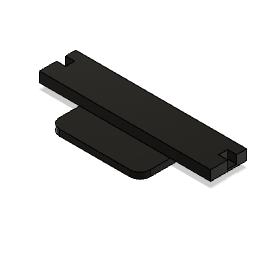
closing_electronic_box (Autodesk Fusion 360 design; units mm, degrees)
Autodesk Fusion 360 part; units mm, degrees
note: some values were not read from the file. Set by a fixed rule: which sketch regions a step uses.
sketch "Esquisse1" plane through (0, 0, 0) normal (0, 1, 0) x (1, 0, 0)
  line L0 (-42.5, 9) -> (42.5, 9)
  line L1 (42.5, 9) -> (42.5, -9)
  line L2 (42.5, -9) -> (-42.5, -9)
  line L3 (-42.5, -9) -> (-42.5, 9)
  line L4 (-42.5, 9) -> (42.5, -9) construction
  line L5 (42.5, 9) -> (-42.5, -9) construction
  dimension "d1" = 18
  dimension "d2" = 85
  constraint horizontal L0
  constraint perpendicular L0 L1
  constraint parallel L0 L2
  constraint parallel L1 L3
  constraint coincident L4 origin
  constraint coincident L5 origin
  measures "d1" distance of L0.start L2.end
  measures "d2" distance of L1.end L2.end
extrude "Extrusion1" add sketch "Esquisse1" along normal blind 5
sketch "Esquisse2" plane through (0, 5, 0) normal (0, 1, 0) x (-1, 0, 0)
  line L0 (42.5, 9) -> (-42.5, 9)
  line L1 (-42.5, 9) -> (-42.5, -9)
  line L2 (-42.5, -9) -> (42.5, -9)
  line L3 (42.5, -9) -> (42.5, 9)
  line L4 (42.5, -4) -> (38, -4)
  line L5 (38, -4) -> (38, 0.5)
  line L6 (38, 0.5) -> (42.5, 0.5)
  line L7 (42.5, 0.5) -> (42.5, -4)
  line L8 (-42.5, -4) -> (-38, -4)
  line L9 (-38, -4) -> (-38, 0.5)
  line L10 (-38, 0.5) -> (-42.5, 0.5)
  line L11 (-42.5, 0.5) -> (-42.5, -4)
  dimension "d5" = 5
  dimension "d6" = 4.5
  dimension "d7" = 4.5
  dimension "d8" = 5
  dimension "d9" = 4.5
  dimension "d10" = 4.5
  constraint horizontal L4
  constraint vertical L5
  constraint horizontal L6
  constraint vertical L7
  constraint coincident L3 L4.start
  constraint horizontal L8
  constraint vertical L9
  constraint horizontal L10
  constraint vertical L11
  constraint coincident L1 L8.start
  measures "d5" distance of L2 L4
  measures "d6" distance of L4.end L5.end
  measures "d7" distance of L5.end L6.end
  measures "d8" distance of L2 L8
  measures "d9" distance of L8.start L8.end
  measures "d10" distance of L8.end L9.end
extrude "Extrusion2" cut sketch "Esquisse2" against normal blind 4 contours L3 L4 L5 L6 L7 | L1 L8 L9 L10 L11
sketch "Esquisse3" plane through (0, 0, 0) normal (0, -1, 0) x (1, 0, 0)
  line L0 (42.5, 9) -> (-42.5, 9)
  line L1 (-42.5, 9) -> (-42.5, -9)
  line L2 (-42.5, -9) -> (42.5, -9)
  line L3 (42.5, -9) -> (42.5, 9)
  line L4 (-15, 5) -> (15, 5)
  line L5 (15, 5) -> (15, -5)
  line L6 (15, -5) -> (-15, -5)
  line L7 (-15, -5) -> (-15, 5)
  line L8 (-15, 5) -> (15, -5) construction
  line L9 (15, 5) -> (-15, -5) construction
  constraint horizontal L4
  constraint perpendicular L4 L5
  constraint parallel L4 L6
  constraint parallel L5 L7
  constraint coincident L8 origin
  constraint coincident L9 origin
sketch "Esquisse5" plane through (0, 5, 0) normal (0, 1, 0) x (-1, 0, 0)
  line L0 (38, 0.5) -> (42.5, 0.5)
  line L1 (42.5, 0.5) -> (42.5, 9)
  line L2 (42.5, 9) -> (-42.5, 9)
  line L3 (-42.5, 9) -> (-42.5, 0.5)
  line L4 (-42.5, 0.5) -> (-38, 0.5)
  line L5 (-38, 0.5) -> (-38, -4)
  line L6 (-38, -4) -> (-42.5, -4)
  line L7 (-42.5, -4) -> (-42.5, -9)
  line L8 (-42.5, -9) -> (42.5, -9)
  line L9 (42.5, -9) -> (42.5, -4)
  line L10 (42.5, -4) -> (38, -4)
  line L11 (38, -4) -> (38, 0.5)
  line L12 (25, -7.5) -> (-25, -7.5)
  line L13 (-25, -7.5) -> (-25, 7.5)
  line L14 (-25, 7.5) -> (25, 7.5)
  line L15 (25, 7.5) -> (25, -7.5)
  line L16 (25, -7.5) -> (-25, 7.5) construction
  line L17 (-25, -7.5) -> (25, 7.5) construction
  dimension "d15" = 15
  dimension "d16" = 50
  constraint horizontal L12
  constraint perpendicular L12 L13
  constraint parallel L12 L14
  constraint parallel L13 L15
  constraint coincident L16 origin
  constraint coincident L17 origin
  measures "d15" distance of L12.start L14.end
  measures "d16" distance of L12.start L12.end
sketch "Esquisse6" plane through (0, 0, 0) normal (0, -1, 0) x (1, 0, 0)
  line L0 (42.5, 9) -> (-42.5, 9)
  line L1 (-42.5, 9) -> (-42.5, -9)
  line L2 (-42.5, -9) -> (42.5, -9)
  line L3 (42.5, -9) -> (42.5, 9)
  line L4 (-17.5, 5) -> (17.5, 5)
  line L5 (20, 2.5) -> (20, -2.5)
  line L6 (17.5, -5) -> (-18, -5)
  line L7 (-20, -3) -> (-20, 2.5)
  line L8 (-20, 5) -> (20, -5) construction
  line L9 (20, 5) -> (-20, -5) construction
  arc A0 (-17.5, 5) -> (-20, 2.5) centre (-17.5, 2.5) ccw
  arc A1 (20, 2.5) -> (17.5, 5) centre (17.5, 2.5) ccw
  arc A2 (17.5, -5) -> (20, -2.5) centre (17.5, -2.5) ccw
  arc A3 (-20, -3) -> (-18, -5) centre (-18, -3) ccw
  dimension "d19" = 2.5
  dimension "d20" = 2
  constraint horizontal L4
  constraint perpendicular L4 L5
  constraint parallel L4 L6
  constraint parallel L5 L7
  constraint coincident L8 origin
  constraint coincident L9 origin
  constraint coincident L8.start L7
  constraint coincident L8.start L4
  constraint tangent L7 A0
  constraint tangent L4 A0
  constraint coincident L9.start L4
  constraint coincident L9.start L5
  constraint tangent L4 A1
  constraint tangent L5 A1
  constraint equal A0 A1
  constraint coincident L8.end L6
  constraint coincident L8.end L5
  constraint tangent L6 A2
  constraint tangent L5 A2
  constraint equal A0 A2
  constraint coincident L9.end L7
  constraint coincident L9.end L6
  constraint tangent L7 A3
  constraint tangent L6 A3
  measures "d19" radius of A0
  measures "d20" radius of A3
sketch "Esquisse7" plane through (0, 0, 0) normal (0, -1, 0) x (1, 0, 0)
  line L0 (42.5, 9) -> (-42.5, 9)
  line L1 (-42.5, 9) -> (-42.5, -9)
  line L2 (-42.5, -9) -> (42.5, -9)
  line L3 (42.5, -9) -> (42.5, 9)
  line L4 (-20, 2.5) -> (20, 2.5)
  line L5 (20, 2.5) -> (20, 5)
  line L6 (20, 5) -> (-20, 5)
  line L7 (-20, 5) -> (-20, 2.5)
  constraint perpendicular L5 L6
extrude "Extrusion6" add sketch "Esquisse7" against normal blind 2 contours L4 L5 L6 L7
sketch "Esquisse8" plane through (0, 0, 0) normal (0, -1, 0) x (1, 0, 0)
  line L0 (42.5, 9) -> (-42.5, 9)
  line L1 (-42.5, 9) -> (-42.5, -9)
  line L2 (-42.5, -9) -> (42.5, -9)
  line L3 (42.5, -9) -> (42.5, 9)
  line L4 (-22.5, 0) -> (22.5, 0)
  line L5 (22.5, 0) -> (22.5, 19)
  line L6 (17.5, 24) -> (-17.5, 24)
  line L7 (-22.5, 19) -> (-22.5, 0)
  arc A0 (-17.5, 24) -> (-22.5, 19) centre (-17.5, 19) ccw
  arc A1 (22.5, 19) -> (17.5, 24) centre (17.5, 19) ccw
  dimension "d25" = 20
  dimension "d26" = 20
  dimension "d27" = 15
  dimension "d28" = 5
  dimension "d29" = 9
  dimension "d30" = 5
  constraint horizontal L4
  constraint vertical L5
  constraint horizontal L6
  constraint vertical L7
  constraint tangent L7 A0
  constraint tangent L6 A0
  constraint tangent L6 A1
  constraint tangent L5 A1
  measures "d25" distance of L3 L5
  measures "d26" distance of L1 L7
  measures "d27" distance of L0 L6
  measures "d28" radius of A0
  measures "d29" distance of L2 L4
  measures "d30" radius of A1
extrude "Extrusion7" add sketch "Esquisse8" along normal blind 3 contours L0 L4 L5 L7 | L0 L5 L6 L7 A0 A1
chamfer "Chanfrein1" distance 3 distance2 3 1 edges at (0, -3, 0) measured on face at (5.8333, -3, 8)
